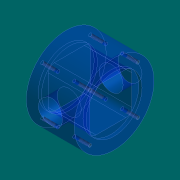
# Autodesk Inventor part: P03
Saved by Autodesk Inventor 2012 SP1 (Build 160190100, 190)
## iProperties
Created: 2011-05-11
Part Number: P03
Material: PVC-U (Transp. / Durchsicht.)
Document SubType Name: Modeling
Designer: sta
Density: 1.4 g/cm^3
Description: Ring
Mass: 23.4854 g
Surface Area: 73.07 cm^2
Volume: 16.7753 cm^3
Title: Kart
Author: sta
Autodesk Inventor part; units mm, degrees
ref_plane "YZ Plane" through (0, 0, 0) normal (1, 0, 0) x (0, 1, 0)
ref_plane "XZ Plane" through (0, 0, 0) normal (0, 1, 0) x (-1, 0, 0)
ref_plane "XY Plane" through (0, 0, 0) normal (0, 0, 1) x (1, 0, 0)
sketch "Sketch1" plane through (0, 0, 0) normal (0, 0, 1) x (1, 0, 0)
  line L0 (-29.3592, 0) -> (29.3592, 0) construction
  line L1 (0, 14.1975) -> (0, -14.1975) construction
  line L2 (-12, 0) -> (12, 0)
  line L3 (12, 0) -> (12, 20)
  line L4 (-12, 20) -> (-12, 0)
  line L5 (-12, 20) -> (-12, 20.8787) construction
  line L6 (12, 20) -> (-12, 20)
  line L7 (50.3592, 10.5) -> (29.3592, 10.5)
  line L8 (29.3592, 10.5) -> (29.3592, -10.5)
  line L9 (29.3592, -10.5) -> (50.3592, -10.5)
  line L10 (50.3592, -10.5) -> (50.3592, 10.5)
  line L11 (29.3592, 0) -> (50.3592, 0) construction
  line L12 (39.8592, 0) -> (39.8592, 3.5595) construction
  circle A0 centre (39.8592, 0) radius 20
  line L13 (33.8592, 10.5) -> (45.8592, 10.5) construction
  line L14 (45.8592, 10.5) -> (45.8592, 24.7953) construction
  line L15 (45.8592, 24.7953) -> (33.8592, 24.7953) construction
  line L16 (33.8592, 24.7953) -> (33.8592, 10.5) construction
  line L17 (33.8592, 18.5) -> (45.8592, 18.5) construction
  point P0 (0, 0)
  point P1 (0, 0)
  point P2 (39.8592, 10.5)
  dimension "d1" = 24
  dimension "d2" = 12
  dimension "d5" = 40
  dimension "d18" = 21
  dimension "d19" = 21
  dimension "d20" = 12
  dimension "d22" = 8
  dimension "d23" = 40
  constraints: 36 end point, 7 midpoint, 7 perpendicular, 5 parallel, 4 horizontal, 4 point on line, 2 coincident, 1 centre point, 1 collinear
  measures "d1" distance between parallel lines of L3 L4
  measures "d2" distance from line of L3 point (0, 0)
  measures "d5" diameter of L6 L0
  measures "d18" distance between parallel lines of L9 L7
  measures "d19" distance between parallel lines of L10 L8
  measures "d20" distance between parallel lines of L14 L16
  measures "d22" distance between parallel lines of L17 L13
  measures "d23" diameter of A0
revolve "Revolution1" add sketch "Sketch1" angle 360 about axis through (-29.3592, 0, 0) along (1, 0, 0) contours L4 L6 L3 L2
sketch "Sketch3" plane through (-12, 0, 0) normal (-1, 0, 0) x (0, 0, 1)
  line L0 (-10.5, 10.5) -> (10.5, 10.5)
  line L1 (10.5, 10.5) -> (10.5, -10.5)
  line L2 (10.5, -10.5) -> (-10.5, -10.5)
  line L3 (-10.5, -10.5) -> (-10.5, 10.5)
  point P0 (0, 0)
  point P1 (0, 10.5)
  point P2 (-10.5, 0)
  dimension "d24" = 21
  dimension "d25" = 21
  constraints: 8 end point, 2 midpoint, 2 parallel, 1 horizontal, 1 horizontal alignment, 1 perpendicular, 1 vertical alignment
  measures "d24" distance between parallel lines of L1 L3
  measures "d25" distance between parallel lines of L2 L0
extrude "Extrusion1" cut sketch "Sketch3" against normal through all
fillet "Fillet1" radius 3 4 edges at (0, 10.5, -10.5) (0, -10.5, -10.5) (0, -10.5, 10.5) (0, 10.5, 10.5)
sketch "Sketch4" plane through (-12, 10.5, -7.5) normal (0, -1, 0) x (1, 0, 0)
  point P0 (12, 7.5)
  point P1 (12, 7.5)
  constraints: 1 coincident
hole "Hole2" at (0, 10.5, 0) direction (0, 1, 0) diameter 12 depth 10 tip angle 118
pattern_circular "Circular Pattern2" count 2 over 360 about axis through (0, 0, 0) along (1, 0, 0) of "Hole2"
sketch "Sketch5" plane through (-12, 0, 0) normal (-1, 0, 0) x (0, 0, 1)
  circle A0 centre (0, 0) radius 14
  dimension "d39" = 28
  constraints: 1 centre point, 1 coincident
  measures "d39" diameter of A0
extrude "Extrusion2" cut sketch "Sketch5" against normal blind 1.6
sketch "Sketch6" plane through (12, 0, 0) normal (1, 0, 0) x (0, 0, -1)
  circle A0 centre (0, 0) radius 14 projected
extrude "Extrusion3" cut sketch "Sketch6" against normal blind 1.6
sketch "Sketch7" plane through (12, 0, 0) normal (1, 0, 0) x (0, 0, -1)
  line L0 (-29.6226, 0) -> (29.6226, 0) construction
  line L1 (0, 0) -> (-16.5524, 16.5524) construction
  circle A0 centre (0, 0) radius 17 construction
  point P0 (-12.0208, 12.0208)
  dimension "d45" = 34
  dimension "d44" = 45
  constraints: 4 end point, 2 coincident, 1 horizontal, 1 midpoint, 1 point on line, 3 other
  measures "d44" angle of L1 L0
hole "Hole3" at (12, 12.0208, 12.0208) direction (-1, 0, 0) diameter 1.567 depth 8 tip angle 118 thread size "M2x0.4" class "6H" standard "ISO Metric profile"
pattern_circular "Circular Pattern3" count 4 over 360 about axis through (0, 0, 0) along (1, 0, 0) of "Hole3"
mirror "Mirror1" about plane through (0, 0, 0) normal (1, 0, 0) of "Hole3", "Circular Pattern3"
equation "\"d2\" = 0.5 * d1"
body "Solid1"
